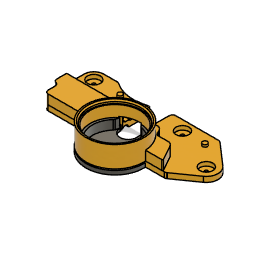
saucer_trackpad_easy_attach (Autodesk Fusion 360 design; units mm, degrees)
Autodesk Fusion 360 part; units mm, degrees
other "Base Mesh Feature1"
other "Modify1"
sketch "Plate - Base shape" plane through (0, 0, 0) normal (0, 1, 0) x (1, 0, 0)
  line L0 (-58.877, 1.3657) -> (-58.877, 32.5256)
  line L1 (-10.5707, 32.5256) -> (-58.877, 32.5256)
  line L2 (-54.8317, -0.5446) -> (-54.8317, -9.2346)
  line L3 (-54.8317, -9.2204) -> (-21.5565, -9.2204)
  line L4 (-10.5707, 32.5256) -> (-10.5707, 8.5256)
  arc A0 (-10.5707, 8.5256) -> (-21.5565, -9.2204) centre (0.4038, -10.5417) ccw
  line L5 (-10.5707, 32.5256) -> (0.59, 32.5256) construction
  line L6 (0.59, 32.5256) -> (0.59, 11.4575)
  line L7 (-56.5009, 1.3657) -> (-58.877, 1.3657)
  line L8 (-56.5009, 1.3657) -> (-54.8317, 1.3657)
  line L9 (-54.8317, 1.3657) -> (-54.8317, -0.5446)
  line L10 (0.59, 32.5256) -> (37.8107, 32.5438)
  line L11 (38.6286, 31.8307) -> (55.9204, 16.7565)
  line L12 (38.6286, 31.8307) -> (37.8107, 32.5438)
  line L13 (38.6137, -8.5762) -> (55.1083, 3.033)
  line L14 (55.1083, 3.033) -> (64.2677, 9.4796)
  line L15 (55.9204, 16.7565) -> (64.2677, 9.4796)
  line L16 (22.3641, -9.2204) -> (37.6985, -9.2204)
  line L17 (38.6137, -8.5762) -> (37.6985, -9.2204)
  circle A1 centre (0.4038, -10.5417) radius 22 construction
  arc A2 (22.3641, -9.2204) -> (0.59, 11.4575) centre (0.4038, -10.5417) ccw
  arc A3 (0.59, 11.4575) -> (-10.5707, 8.5256) centre (0.4038, -10.5417) ccw
  line L18 (-10.5707, 32.5256) -> (0.59, 32.5256)
  line L19 (-21.5565, -9.2204) -> (22.3641, -9.2204)
  point P0 (-56.5269, 8.7841)
  point P1 (-54.8317, -0.5446)
  point P2 (-54.8317, -9.2346)
  point P3 (-54.8317, -9.2204)
  point P4 (-50.3244, 26.0765)
  point P5 (-50.1685, 24.1831)
  point P6 (-49.8696, 25.4516)
  point P7 (-16.0834, 4.0245)
  point P8 (-11.6984, 7.8305)
  point P9 (-56.5009, 1.3657)
  point P10 (38.6286, 31.8307)
  point P11 (38.6137, -8.5762)
  point P12 (55.1083, 3.033)
  dimension "d1" = 24
  dimension "d4" = 22
  constraint horizontal L1
  constraint vertical L0
  constraint coincident P1 L2.start
  constraint coincident P2 L2.end
  constraint vertical L2
  constraint coincident P3 L3.start
  constraint coincident L3.end A0.end
  constraint parallel L1 L3
  constraint coincident P7 A0
  constraint coincident P8 A0
  constraint perpendicular L1 L4
  constraint horizontal L5
  constraint vertical L0.end L1.end
  constraint coincident L0.end L1.end
  constraint coincident P9 L7.start
  constraint perpendicular L0 L7
  constraint coincident L0.start L7.end
  constraint horizontal L8
  constraint vertical L9
  constraint coincident L7 P9
  constraint vertical P2 P3
  constraint coincident P10 L11.start
  constraint collinear L11 L12
  constraint coincident P11 L13.start
  constraint coincident P12 L13.end
  constraint collinear L13 L14
  constraint collinear L11 L15
  constraint horizontal L16
  constraint parallel L13 L17
  constraint collinear L3 L16
  constraint concentric A0 A1
  constraint coincident L3.end A1
  constraint coincident A1 L16.start
  constraint coincident A1 L6.end
  constraint coincident A0.centre A1.centre
  constraint perpendicular L6 L18
  measures "d1" distance of L1.start L4.end
  measures "d4" radius of A0
extrude "Extrude1" add sketch "Plate - Base shape" against normal blind 4 makes body 1
fillet "Fillet1" radius 9 1 edges at (64.2677, -2, -9.4796) on bodies 1
fillet "Fillet3" radius 7.5 1 edges at (-58.877, -2, -32.5256) on bodies 1
fillet "Fillet5" radius 2.5 4 edges at (-54.8317, -2, 9.2204) (-58.877, -2, -1.3657) (37.6985, -2, 9.2204) (37.8107, -2, -32.5438) on bodies 1
fillet "Fillet5" radius 2.5 1 edges at (-54.8317, -2, -1.3657) on bodies 1
sketch "Plate - Tube base shape" plane through (0, 0, 0) normal (0, 1, 0) x (1, 0, 0)
  circle A0 centre (0.4817, -10.6186) radius 19.2993
  circle A1 centre (0.4038, -10.5417) radius 22
  point P0 (-10.5769, 5.1981)
  point P1 (-13.3264, -24.1019)
  point P2 (19.6138, -13.1535)
  constraint coincident P0 A0
  constraint coincident P1 A0
  constraint coincident P2 A0
sketch "Plate - Voyager edge align" plane through (0, 0, 0) normal (0, 1, 0) x (1, 0, 0)
  line L0 (-58.88, 11.6027) -> (10.8429, 11.6027)
  arc A0 (14.1275, 9.745) -> (10.8429, 11.6027) centre (10.7587, 7.6212) ccw
  arc A1 (15.22, 7.8) -> (14.1275, 9.745) centre (2.5732, 1.9757) ccw
  arc A2 (16.2489, 6.0211) -> (17.7811, 5.2368) centre (17.794, 7.1507) ccw
  arc A3 (15.6277, 6.9909) -> (16.2489, 6.0211) centre (21.7446, 10.2255) ccw
  arc A4 (15.22, 7.8) -> (15.6277, 6.9909) centre (31.1534, 15.3213) ccw
  arc A5 (28.9825, 3.2225) -> (25.5193, 5.2467) centre (25.4378, 1.1326) ccw
  line L1 (17.7811, 5.2368) -> (25.5193, 5.2467)
  line L2 (28.9825, 3.2225) -> (35.4595, -8.4085)
  line L3 (35.4595, -8.4085) -> (35.9116, -9.2204)
  arc A6 (-54.8317, -1.0423) -> (-56.8543, 1.4117) centre (-57.3317, -1.0423) ccw
  line L4 (-54.8317, -1.0423) -> (-54.8317, -6.7204)
  arc A7 (-58.877, 3.8657) -> (-56.8543, 1.4117) centre (-56.377, 3.8657) ccw
  line L5 (-58.877, 3.8657) -> (-58.88, 11.6027)
  arc A8 (-54.8317, -6.7204) -> (-52.3317, -9.2204) centre (-52.3317, -6.7204) ccw
  line L6 (-52.3317, -9.2204) -> (35.9116, -9.2204)
  line L7 (-52.3317, -9.2204) -> (36.907, -9.2204)
  point P0 (15.22, 7.8)
  point P1 (17.7811, 5.2368)
  point P2 (14.1275, 9.745)
  point P3 (16.2489, 6.0211)
  point P4 (15.6277, 6.9909)
  point P5 (25.5193, 5.2467)
  point P6 (28.9825, 3.2225)
  point P7 (35.4595, -8.4085)
  constraint horizontal L0
  constraint coincident P2 A0.start
  constraint coincident L0.end A0.end
  constraint coincident P0 A1.start
  constraint coincident P3 A2.start
  constraint coincident P1 A2.end
  constraint coincident P4 A3.start
  constraint coincident P6 A5.start
  constraint coincident P5 A5.end
  constraint coincident P7 L2.end
  constraint collinear L2 L3
  constraint collinear L6 L7
extrude "Extrude2" add sketch "Plate - Voyager edge align" along normal blind 7.2 bodies 1
sketch "Plate - Bottom align nubs" plane through (0, 0, 0) normal (0, 1, 0) x (1, 0, 0)
  circle A0 centre (-30.2075, 24.0382) radius 1.875
  circle A1 centre (34.7911, 24.1216) radius 1.875
  point P0 (-31.5166, 25.3806)
  point P1 (-28.3462, 24.2639)
  point P2 (-30.7879, 22.2553)
  dimension "d26" = 3.75
  constraint coincident P0 A0
  constraint coincident P1 A0
  constraint coincident P2 A0
  constraint equal A0 A1
  measures "d26" diameter of A0
extrude "Extrude3" add sketch "Plate - Bottom align nubs" along normal blind 1.6 bodies 1
fillet "Fillet6" radius 0.55 1 edges at (35.9116, 3.6, 9.2204) on bodies 1
sketch "Plate - Magnet holes" plane through (0, 0, 0) normal (0, 1, 0) x (-1, 0, 0)
  circle A0 centre (30.2075, -24.0382) radius 1.875
  circle A1 centre (-34.7911, -24.1216) radius 1.875
  line L0 (58.877, -11.6027) -> (-10.8429, -11.6027)
  arc A2 (-14.1275, -9.745) -> (-10.8429, -11.6027) centre (-10.7587, -7.6212) ccw
  arc A3 (-15.22, -7.8) -> (-14.1275, -9.745) centre (-2.5732, -1.9757) ccw
  arc A4 (-15.22, -7.8) -> (-15.6277, -6.9909) centre (-31.1534, -15.3213) ccw
  arc A5 (-15.6277, -6.9909) -> (-16.2489, -6.0211) centre (-21.7446, -10.2255) ccw
  arc A6 (-16.2489, -6.0211) -> (-17.7811, -5.2368) centre (-17.794, -7.1507) ccw
  line L1 (-17.7811, -5.2368) -> (-25.5193, -5.2467)
  arc A7 (-28.9825, -3.2225) -> (-25.5193, -5.2467) centre (-25.4378, -1.1326) ccw
  line L2 (-28.9825, -3.2225) -> (-35.4563, 8.4028)
  arc A8 (-34.9758, 9.2204) -> (-35.4563, 8.4028) centre (-34.9758, 8.6704) ccw
  line L3 (-34.9758, 9.2204) -> (-35.9116, 9.2204)
  arc A9 (-36.907, 9.2204) -> (-38.3459, 8.7648) centre (-36.907, 6.7204) ccw
  line L4 (-38.3459, 8.7648) -> (-38.6137, 8.5762)
  line L5 (-38.6137, 8.5762) -> (-54.8846, -2.8756)
  arc A10 (-54.8846, -2.8756) -> (-55.6187, -17.0195) centre (-49.7046, -10.2354) ccw
  line L6 (-55.6187, -17.0195) -> (-38.5173, -31.9278)
  arc A11 (-38.5173, -31.9278) -> (-36.8733, -32.5433) centre (-36.8745, -30.0433) ccw
  line L7 (-36.8733, -32.5433) -> (-0.59, -32.5256)
  line L8 (-0.59, -32.5256) -> (51.377, -32.5256)
  arc A12 (51.377, -32.5256) -> (58.877, -25.0256) centre (51.377, -25.0256) ccw
  line L9 (58.877, -25.0256) -> (58.877, -11.6027)
  arc A13 (-54.8846, -2.8756) -> (-55.6187, -17.0195) centre (-49.7046, -10.2354) ccw construction
  arc A14 (51.377, -32.5256) -> (58.877, -25.0256) centre (51.377, -25.0256) ccw construction
  circle A15 centre (-49.7046, -10.2354) radius 5
  circle A16 centre (51.377, -25.0256) radius 5
  line L10 (58.877, -25.0256) -> (-46.4349, -25.0256) construction
  circle A17 centre (-16.6447, -25.0256) radius 5
  circle A18 centre (19.167, -20.0256) radius 5
  circle A19 centre (-49.7046, -10.2354) radius 1.25
  circle A20 centre (-16.6447, -25.0256) radius 1.25
  circle A21 centre (19.167, -20.0256) radius 1.25
  circle A22 centre (51.377, -25.0256) radius 1.25
  line L11 (-35.9116, 9.2204) -> (-36.907, 9.2204)
  line L12 (19.167, -18) -> (19.167, -32.5256) construction
  dimension "d31" = 10
  dimension "d34" = 2.5
  constraint concentric A13 A15
  constraint concentric A14 A16
  constraint equal A15 A16
  constraint coincident L6 L10.end
  constraint horizontal L10
  constraint coincident L10 A17.centre
  constraint equal A17 A18
  constraint equal A15 A17
  constraint concentric A13 A19
  constraint concentric A17 A20
  constraint concentric A18 A21
  constraint concentric A16 A22
  constraint equal A19 A20
  constraint equal A20 A21
  constraint equal A21 A22
  constraint coincident L8 L12.end
  constraint perpendicular L8 L12
  measures "d31" diameter of A15
  measures "d34" diameter of A19
extrude "Extrude4" cut sketch "Plate - Magnet holes" against normal blind 3 contours A15 | A16 | A17 | A18 | A19 | A20 | A21 | A22 bodies 1
extrude "Extrude5" cut sketch "Plate - Magnet holes" against normal up to surface (4 mm away) contours A19 | A20 | A21 | A22 bodies 1
sketch "Plate - Sensor housing tube" plane through (0, 0, 0) normal (0, 1, 0) x (1, 0, 0)
  circle A0 centre (0.4038, -10.5417) radius 22 construction
  circle A1 centre (0.4038, -10.5417) radius 19.9 construction
  circle A2 centre (0.4038, -10.5417) radius 19.1
  circle A3 centre (0.4038, -10.5417) radius 22.1354
  arc A4 (15.6277, 6.9909) -> (16.2489, 6.0211) centre (21.7446, 10.2255) ccw
  arc A5 (16.2489, 6.0211) -> (17.7811, 5.2368) centre (17.794, 7.1507) ccw
  arc A6 (15.22, 7.8) -> (14.1275, 9.745) centre (2.5732, 1.9757) ccw
  arc A7 (15.22, 7.8) -> (15.6277, 6.9909) centre (31.1534, 15.3213) ccw
  arc A8 (14.1275, 9.745) -> (10.8429, 11.6027) centre (10.7587, 7.6212) ccw
  line L0 (10.8429, 11.6027) -> (-58.88, 11.6027)
  line L1 (25.5193, 5.2467) -> (17.7811, 5.2368)
  dimension "d37" = 39.8
  dimension "d38" = 0.8
  constraint concentric A0 A1
  constraint concentric A0 A2
  constraint concentric A2 A3
  measures "d37" diameter of A1
  measures "d38" distance of A1 A2
extrude "Extrude6" add sketch "Plate - Sensor housing tube" along normal blind 15 bodies 1
extrude "Extrude7" cut sketch "Plate - Sensor housing tube" along normal up to surface (-4 mm away) and the other way up to surface (-7.2 mm away) contours A2 bodies 1
sketch "Plate - Sensor housing cutout" plane through (0, 15, 0) normal (0, 1, 0) x (-1, 0, 0)
  circle A0 centre (-0.4038, 10.5417) radius 19.1
  circle A1 centre (-0.4038, 10.5417) radius 22.1354
  circle A2 centre (-0.4038, 10.5417) radius 20
  circle A3 centre (-0.4038, 10.5417) radius 19.2
extrude "Extrude8" cut sketch "Plate - Sensor housing cutout" against normal blind 1.3 contours A2 | A3 bodies 1
sketch "Plate - Sensor housing lid cutout" plane through (0, -4, 0) normal (0, -1, 0) x (1, 0, 0)
  arc A0 (-18.6505, 9.2204) -> (19.458, 9.2204) centre (0.4038, 10.5417) ccw
  line L0 (-18.6505, 9.2204) -> (-52.3317, 9.2204)
  arc A1 (-52.3317, 9.2204) -> (-54.8317, 6.7204) centre (-52.3317, 6.7204) ccw
  line L1 (-54.8317, 6.7204) -> (-54.8317, 1.0423)
  arc A2 (-56.8543, -1.4117) -> (-54.8317, 1.0423) centre (-57.3317, 1.0423) ccw
  arc A3 (-56.8543, -1.4117) -> (-58.877, -3.8657) centre (-56.377, -3.8657) ccw
  line L2 (-58.877, -3.8657) -> (-58.877, -25.0256)
  arc A4 (-58.877, -25.0256) -> (-51.377, -32.5256) centre (-51.377, -25.0256) ccw
  line L3 (-51.377, -32.5256) -> (0.59, -32.5256)
  line L4 (0.59, -32.5256) -> (36.8733, -32.5433)
  arc A5 (36.8733, -32.5433) -> (38.5173, -31.9278) centre (36.8745, -30.0433) ccw
  line L5 (38.5173, -31.9278) -> (55.6187, -17.0195)
  arc A6 (55.6187, -17.0195) -> (54.8846, -2.8756) centre (49.7046, -10.2354) ccw
  line L6 (54.8846, -2.8756) -> (38.6137, 8.5762)
  line L7 (38.6137, 8.5762) -> (38.3459, 8.7648)
  arc A7 (38.3459, 8.7648) -> (36.907, 9.2204) centre (36.907, 6.7204) ccw
  line L8 (36.907, 9.2204) -> (19.458, 9.2204)
  circle A8 centre (-51.377, -25.0256) radius 1.25
  circle A9 centre (49.7046, -10.2354) radius 1.25
  circle A10 centre (-19.167, -20.0256) radius 1.25
  circle A11 centre (16.6447, -25.0256) radius 1.25
  circle A12 centre (0.4038, 10.5417) radius 20.1
  dimension "d47" = 1
  constraint concentric A0 A12
  measures "d47" distance of A0 A12
extrude "Extrude9" cut sketch "Plate - Sensor housing lid cutout" against normal up to surface (4 mm away) contours A0 L0 L8 A12 picked at (-19.1872, 8.2699) bodies 1
sketch "Plate - Cable installation gap" plane through (0, -4, 0) normal (0, -1, 0) x (1, 0, 0)
  circle A0 centre (16.6447, -25.0256) radius 1.25
  circle A1 centre (-19.167, -20.0256) radius 1.25
  circle A2 centre (49.7046, -10.2354) radius 1.25
  circle A3 centre (-51.377, -25.0256) radius 1.25
  arc A4 (-19.6528, 9.2204) -> (20.4603, 9.2204) centre (0.4038, 10.5417) ccw
  line L0 (-19.6528, 9.2204) -> (-52.3317, 9.2204)
  arc A5 (-52.3317, 9.2204) -> (-54.8317, 6.7204) centre (-52.3317, 6.7204) ccw
  line L1 (-54.8317, 6.7204) -> (-54.8317, 1.0423)
  arc A6 (-56.8543, -1.4117) -> (-54.8317, 1.0423) centre (-57.3317, 1.0423) ccw
  arc A7 (-56.8543, -1.4117) -> (-58.877, -3.8657) centre (-56.377, -3.8657) ccw
  line L2 (-58.877, -3.8657) -> (-58.877, -25.0256)
  arc A8 (-58.877, -25.0256) -> (-51.377, -32.5256) centre (-51.377, -25.0256) ccw
  line L3 (-51.377, -32.5256) -> (0.59, -32.5256)
  line L4 (0.59, -32.5256) -> (36.8733, -32.5433)
  arc A9 (36.8733, -32.5433) -> (38.5173, -31.9278) centre (36.8745, -30.0433) ccw
  line L5 (38.5173, -31.9278) -> (55.6187, -17.0195)
  arc A10 (55.6187, -17.0195) -> (54.8846, -2.8756) centre (49.7046, -10.2354) ccw
  line L6 (54.8846, -2.8756) -> (38.6137, 8.5762)
  line L7 (38.6137, 8.5762) -> (38.3459, 8.7648)
  arc A11 (38.3459, 8.7648) -> (36.907, 9.2204) centre (36.907, 6.7204) ccw
  line L8 (36.907, 9.2204) -> (20.4603, 9.2204)
  line L9 (-10.5962, -6.2812) -> (-10.5962, -32.5256)
  line L10 (1.4038, -32.5348) -> (-10.5962, -32.5256)
  arc A12 (-10.5962, -5.0614) -> (1.4038, -8.3934) centre (0.3577, 11.1137) ccw
  line L11 (-11.6467, -4.2631) -> (-12.274, -5.0559)
  arc A13 (-11.6467, -4.2631) -> (-10.5962, -5.0614) centre (-3.4375, 5.4483) ccw
  arc A14 (-12.274, -5.0559) -> (-10.5962, -6.2812) centre (0.4038, 10.5417) ccw
  line L12 (1.4038, -8.3934) -> (1.4038, -32.5348)
  dimension "d89" = 12
  constraint coincident A4 L9.start
  constraint coincident L3 L9.end
  constraint perpendicular L3 L9
  constraint coincident A4 L11.end
  constraint vertical L10.start A12.end
  measures "d89" horizontal distance of L10.start L9.end
extrude "Extrude13" cut sketch "Plate - Cable installation gap" against normal blind 9.791 contours A4 A12 L11 A13 A14 L12 | A4 L3 L4 L9 L12 bodies 1
sketch "Plate - Bottom cable guide" plane through (-58.877, 0, 0) normal (-1, 0, 0) x (0, 0, 1)
  line L0 (-3.8657, -4) -> (-3.8657, 0)
  line L1 (-3.8657, 0) -> (-11.6027, 0)
  line L2 (-11.6027, 0) -> (-25.0256, 0)
  line L3 (-25.0256, 0) -> (-25.0256, -4)
  line L4 (-25.0256, -4) -> (-3.8657, -4)
  line L5 (-3.8657, 0) -> (-10.9249, 0) construction
  line L6 (-10.9249, 0) -> (-10.9249, -4) construction
  line L7 (-10.9249, -4) -> (-3.8657, -4) construction
  line L8 (-3.8657, -4) -> (-3.8657, 0) construction
  line L9 (-11.6027, 0) -> (-11.6027, 7.2) construction
  line L10 (-11.6027, 0) -> (-5.9249, -4) construction
  line L11 (-10.9249, -4) -> (-5.9249, 0) construction
  line L12 (-5.9249, 0) -> (-5.9249, -4) construction
  line L13 (-10.9249, -4) -> (-10.9249, -3.5907)
  line L14 (-5.9249, -4) -> (-5.9249, -3.5907)
  line L15 (-10.9249, -3.5907) -> (-5.9249, -3.5907) construction
  line L16 (-5.9249, -3.5907) -> (-5.9249, -1.6)
  line L17 (-5.9249, -1.6) -> (-10.9249, -1.6)
  line L18 (-10.9249, -1.6) -> (-10.9249, -3.5907)
  dimension "d85" = 1.6
  dimension "d93" = 5
  constraint horizontal L5
  constraint vertical L6
  constraint horizontal L7
  constraint vertical L8
  constraint coincident L4 L6.end
  constraint coincident L0.end L1.start
  constraint coincident L1.end L2.start
  constraint coincident L7 L10.end
  constraint coincident L5 L11.end
  constraint vertical L12
  constraint coincident L6 L13.end
  constraint coincident L12 L14.end
  constraint horizontal L13.end L14.end
  constraint horizontal L15
  constraint vertical L16
  constraint horizontal L17
  constraint vertical L18
  constraint coincident L12 L16.end
  measures "d85" distance of L5 L17
  measures "d93" distance of L16.end L17.end
extrude "Extrude14" cut sketch "Plate - Bottom cable guide" against normal blind 51 contours L4 L13 L14 L16 L17 L18 bodies 1
fillet "Fillet8" radius 2.5 2 edges at (-34.7366, -1.6, -10.9249) (-34.9999, -1.6, -5.9249) on bodies 1
sketch "Plate - Top cable guide" plane through (-58.8755, 0, 0.0228) normal (-1, 0, 0.000387) x (0.000387, 0, 1)
  line L0 (-11.6255, 0) -> (-3.8885, 0)
  line L1 (-3.8885, 0) -> (-3.8885, 7.2)
  line L2 (-3.8885, 7.2) -> (-11.6255, 7.2)
  line L3 (-11.6255, 7.2) -> (-11.6255, 0)
  line L4 (-11.6255, 4.8) -> (-8.4497, 4.8)
  arc A0 (-8.4497, 0.8) -> (-8.4497, 4.8) centre (-8.4497, 2.8) ccw
  line L5 (-8.4497, 0.8) -> (-11.6255, 0.8)
  line L6 (-11.6255, 0.8) -> (-11.6255, 4.8)
  point P0 (-6.4497, 2.8)
  point P1 (-8.4497, -1.6)
  dimension "d96" = 2.4
  dimension "d97" = 2
  constraint coincident L3 L4.start
  constraint perpendicular L3 L4
  constraint tangent L4 A0
  constraint vertical L4.end A0.start
  constraint midpoint A0 P0
  constraint vertical A0.start P1
  constraint coincident L3 L5.end
  constraint tangent A0 L5
  constraint perpendicular L3 L5
  measures "d96" distance of A0.start P1
  measures "d97" radius of A0
sketch "Lid - Inner compartment" plane through (0, 0, 0) normal (0, -1, 0) x (1, 0, 0)
  line L0 (1.4038, -8.5321) -> (1.4038, -9.5334)
  arc A0 (1.4038, -9.5334) -> (20.4603, 9.2204) centre (0.4038, 10.5417) ccw
  line L1 (20.4603, 9.2204) -> (22.4997, 9.2204)
  arc A1 (22.4997, 9.2204) -> (-21.6921, 9.2204) centre (0.4038, 10.5417) ccw
  line L2 (-21.6921, 9.2204) -> (-19.6528, 9.2204)
  arc A2 (-19.6528, 9.2204) -> (-12.274, -5.0559) centre (0.4038, 10.5417) ccw
  line L3 (-12.274, -5.0559) -> (-11.6534, -4.2716)
  arc A3 (1.4038, -8.5321) -> (-11.6534, -4.2716) centre (0.4038, 10.5417) ccw
  circle A4 centre (0.4038, 10.5417) radius 19.1
  circle A5 centre (0.4038, 10.5417) radius 19.9
  line L4 (20.2722, 9.4208) -> (22.5108, 9.4208)
  line L5 (20.2599, 9.2204) -> (20.4603, 9.2204) construction
  line L6 (20.4603, 9.2204) -> (20.4603, 9.4208) construction
  line L7 (-19.4646, 9.4208) -> (-21.7032, 9.4208)
  arc A6 (22.5108, 9.4208) -> (-21.7032, 9.4208) centre (0.4038, 10.5417) ccw
  line L8 (1.4038, -8.5321) -> (1.4038, -4.8861)
  line L9 (-11.1228, -5.6802) -> (-11.1228, -4.8861)
  arc A7 (1.4038, -4.8861) -> (-11.1228, -4.8861) centre (-4.8595, -4.8861) ccw
  point P0 (-11.1228, -5.9249)
  dimension "d98" = 0.2
  constraint concentric A0 A4
  constraint concentric A4 A5
  constraint equal A3 A4
  constraint coincident A5 L4.start
  constraint coincident A1 L4.end
  constraint horizontal L4
  constraint coincident A5 L5.start
  constraint coincident A0.end L1.start
  constraint horizontal L5
  constraint coincident L4 L6.end
  constraint perpendicular L4 L6
  constraint equal L5 L6
  constraint coincident A5 L7.start
  constraint coincident A1 L7.end
  constraint horizontal L7
  constraint collinear L4 L7
  constraint coincident L0.start A3.start
  constraint parallel L0 L8
  constraint coincident A5 L9.start
  constraint parallel L8 L9
  constraint vertical L9.start P0
  constraint horizontal L8.end L9.end
  constraint tangent L9 A7
  measures "d98" distance of A2 A5
extrude "Extrude15" add sketch "Lid - Inner compartment" against normal blind 5 separate body contours A3 A4 L8 A7 makes body 2
extrude "Extrude17" add sketch "Lid - Inner compartment" along normal up to surface (4 mm away) separate body contours L0 L3 A3 A4 A5 | A3 A4 L8 A7 | L3 A4 A5 L9 A7 | A1 A5 L4 L7 A6 makes body 3
combine "Combine1" operation add target body 2 tool bodies 3
extrude "Extrude19" cut sketch "Plate - Top cable guide" along normal up to surface contours L3 L4 A0 L5 L6 end surface through (-10.5962, -4, -6.2812) normal (1, 0, 0) offset 0 bodies 1
sketch "lid hole (1)" plane through (0, 5, 0) normal (0, 1, 0) x (-1, 0, 0)
  line L0 (-1.4038, -8.5321) -> (-1.4038, -4.8861)
  arc A0 (11.1197, -4.6905) -> (-1.4038, -4.8861) centre (4.8595, -4.8861) ccw
  line L1 (11.1197, -4.6905) -> (12.1247, -1.3884)
  line L2 (-3.2038, -6.5302) -> (-1.4038, -8.5321)
  arc A1 (11.1197, -4.6905) -> (-1.4038, -8.5321) centre (-0.4038, 10.5417) ccw
  arc A2 (12.1247, -1.3884) -> (-3.2038, -4.8861) centre (4.8595, -4.8861) ccw
  line L3 (-3.2038, -6.5302) -> (-3.2038, -4.8861)
  arc A3 (12.1247, -1.3884) -> (-3.2038, -6.5302) centre (-0.4038, 10.5417) ccw
  dimension "d107" = -1.8
  constraint coincident A0.start L1.start
  constraint coincident L0.start L2.end
extrude "lid hole" cut sketch "lid hole (1)" against normal blind 7 contours L0 A0 L1 L2 A2 L3 | A2 L3 A3 bodies 2
sketch "Plate - Magnetic stand cutout" plane through (0, 0, 0) normal (0, 1, 0) x (1, 0, 0)
  line L0 (5.2197, 55.3086) -> (-51.5023, 55.3086) construction
  circle A0 centre (-23.1413, 55.3086) radius 28.361
  constraint horizontal L0
  constraint midpoint L0 A0.centre
  constraint coincident L0.start A0
extrude "Extrude20" cut sketch "Plate - Magnetic stand cutout" against normal blind 4 bodies 1
fillet "Fillet9" radius 2.5 2 edges at (-10.5962, -2, -29.873) (-40.0316, -2, -32.5256) on bodies 1
fillet "Fillet9" radius 2.5 1 edges at (1.4038, -2, -32.526) on bodies 1
fillet "Fillet10" radius 2.5 2 edges at (3.2038, 1.5, -6.5302) (-12.1247, 1.5, -1.3884) on bodies 2
sketch "Plate - Plane guide for Sensor scroll edge" plane through (0, 15, 0) normal (0, 1, 0) x (-1, 0, 0)
  circle A0 centre (-0.4038, 10.5417) radius 20
  circle A1 centre (-0.4038, 10.5417) radius 22.1354
  circle A2 centre (-0.4038, 10.5417) radius 20 construction
  line L0 (-0.4038, 10.5417) -> (-29.4305, 10.5417) construction
  line L1 (-0.4038, 10.5417) -> (29.4863, 10.5417) construction
  constraint coincident A0.centre A1.centre
  constraint horizontal L0
  constraint parallel L0 L1
ref_plane "WorkPlane3" through (-37.0119, 3.6, 9.2204) normal (0, 0, 1) x (1, 0, 0)
ref_plane "WorkPlane4" through (28.7377, 3.6, 10.5417) normal (0, 0, 1) x (1, 0, 0)
sketch "Plate - Sensor scroll edge" plane through (0, 0, 10.5417) normal (0, 0, 1) x (1, 0, 0)
  line L0 (22.5392, 15) -> (-21.7316, 15)
  line L1 (20.4038, 15) -> (-19.5962, 15)
  line L2 (0.4038, 15) -> (0.4038, 43) construction
  line L3 (-21.7316, 15) -> (-21.7316, 16.2)
  line L4 (-21.7316, 16.2) -> (-20.5316, 16.2)
  line L5 (-20.5316, 16.2) -> (-19.5962, 15)
  dimension "d151" = 1.2
  dimension "d152" = 1.2
  constraint midpoint L1 L2.start
  constraint perpendicular L1 L2
  constraint coincident L0.end L3.start
  constraint parallel L0 L4
  constraint coincident L1.end L5.end
  constraint vertical L3
  measures "d151" distance of L3.end L4.end
  measures "d152" distance of L0 L4
revolve "Revolve1" add sketch "Plate - Sensor scroll edge" angle 360 about axis through (0.4038, 15, 10.5417) along (0, 1, 0) bodies 1
sketch "Plate - Lid seam hide gap" plane through (0, 0, 0) normal (0, 1, 0) x (-1, 0, 0)
  arc A0 (11.1197, -4.6905) -> (-1.4038, -8.5321) centre (-0.4038, 10.5417) ccw
  arc A1 (11.1228, -4.8861) -> (11.1197, -4.6905) centre (4.8595, -4.8861) ccw
  line L0 (11.1228, -4.8861) -> (11.1228, -5.6802)
  arc A2 (11.1228, -5.6802) -> (19.4646, 9.4208) centre (-0.4038, 10.5417) ccw
  line L1 (19.4646, 9.4208) -> (21.7032, 9.4208)
  arc A3 (21.7032, 9.4208) -> (-22.5108, 9.4208) centre (-0.4038, 10.5417) ccw
  line L2 (-22.5108, 9.4208) -> (-20.2722, 9.4208)
  arc A4 (-20.2722, 9.4208) -> (-1.4038, -9.3332) centre (-0.4038, 10.5417) ccw
  line L3 (-1.4038, -9.3332) -> (-1.4038, -8.5321)
  circle A5 centre (-0.4038, 10.5417) radius 19.9
  constraint coincident A2.end A5
  constraint coincident L2.end A5
  constraint coincident L0.end A5
extrude "Extrude22" cut sketch "Plate - Lid seam hide gap" against normal blind 1 contours L1 A3 L2 A5 bodies 2
named bodies: "Saucer_trackpad_easy_attach_plate_RIGHT", "Saucer_trackpad_easy_attach_lid_RIGHT (1)"
